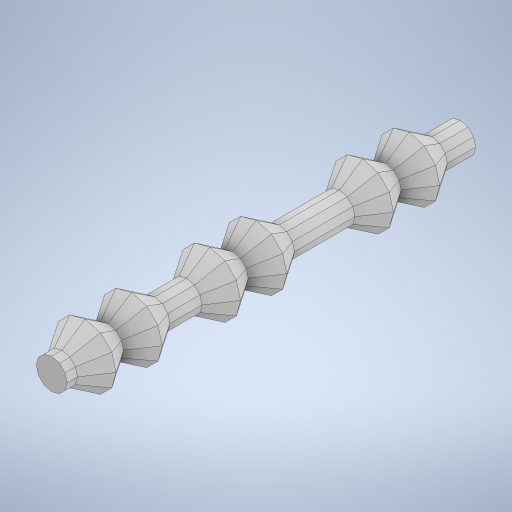
# Autodesk Inventor part: Finger
Saved by Autodesk Inventor 2023 (Build 270158000, 158)
## iProperties
Created: 2024-07-10
Part Number: Finger
Material: 일반
Document SubType Name: Modeling
Designer: ojs08
Density: 1 g/cm^3
Appearance: 기본값
Author: ojs08
Autodesk Inventor part; units mm, degrees
sketch "스케치1" plane through (0, 0, 0) normal (0, 0, 1) x (1, 0, 0)
  line L0 (6, -10.392305) -> (0, -12)
  line L1 (0, -12) -> (-6, -10.392305)
  line L2 (-6, -10.392305) -> (-10.392305, -6)
  line L3 (-10.392305, -6) -> (-12, 0)
  line L4 (-12, 0) -> (-10.392305, 6)
  line L5 (-10.392305, 6) -> (-6, 10.392305)
  line L6 (-6, 10.392305) -> (0, 12)
  line L7 (0, 12) -> (6, 10.392305)
  line L8 (6, 10.392305) -> (10.392305, 6)
  line L9 (10.392305, 6) -> (12, 0)
  line L10 (12, 0) -> (10.392305, -6)
  line L11 (10.392305, -6) -> (6, -10.392305)
  line L12 (-16.8, 0) -> (16.8, 0)
  point P0 (0, 0)
  point P1 (0, 0)
  dimension "d0" = 24
  constraints: 24 end point, 1 coincident, 1 point on line, 25 other
  measures "d0" distance of L9.end L3.end
ref_plane "작업 평면1" through (0, 0, 9) normal (0, 0, 1) x (1, 0, 0)
sketch "스케치2" plane through (0, 0, 9) normal (0, 0, 1) x (1, 0, 0)
  line L0 (-16.8, 0) -> (16.8, 0)
  line L1 (5.196152, -3) -> (3, -5.196152)
  line L2 (3, -5.196152) -> (0, -6)
  line L3 (0, -6) -> (-3, -5.196152)
  line L4 (-3, -5.196152) -> (-5.196152, -3)
  line L5 (-5.196152, -3) -> (-6, 0)
  line L6 (-6, 0) -> (-5.196152, 3)
  line L7 (-5.196152, 3) -> (-3, 5.196152)
  line L8 (-3, 5.196152) -> (0, 6)
  line L9 (0, 6) -> (3, 5.196152)
  line L10 (3, 5.196152) -> (5.196152, 3)
  line L11 (5.196152, 3) -> (6, 0)
  line L12 (6, 0) -> (5.196152, -3)
  point P0 (0, 0)
  point P1 (0, 0)
  dimension "d2" = 12
  constraints: 24 end point, 1 coincident, 1 point on line, 25 other
  measures "d2" distance of L11.end L5.end
loft "로프트1" add profiles "스케치2", "스케치1"
mirror "미러1" about plane through (0, 0, 0) normal (0, 0, -1) of "로프트1"
mirror "미러2" about plane through (0, 0, 9) normal (0, 0, 1) of "로프트1", "미러1"
sketch "스케치3" plane through (3, -5.196152, 27) normal (0, 0, 1) x (0.7071068, -0.7071068, 0)
  line L0 (0, 3.105829) -> (0, 0)
  line L1 (-1.552914, 5.795555) -> (0, 3.105829)
  line L2 (-4.242641, 7.348469) -> (-1.552914, 5.795555)
  line L3 (-7.348469, 7.348469) -> (-4.242641, 7.348469)
  line L4 (-10.038196, 5.795555) -> (-7.348469, 7.348469)
  line L5 (-11.59111, 3.105829) -> (-10.038196, 5.795555)
  line L6 (-11.59111, 0) -> (-11.59111, 3.105829)
  line L7 (-10.038196, -2.689726) -> (-11.59111, 0)
  line L8 (-7.348469, -4.242641) -> (-10.038196, -2.689726)
  line L9 (-4.242641, -4.242641) -> (-7.348469, -4.242641)
  line L10 (-1.552914, -2.689726) -> (-4.242641, -4.242641)
  line L11 (0, 0) -> (-1.552914, -2.689726)
  point P0 (-5.795555, 1.552914)
extrude "돌출1" add sketch "스케치3" along normal blind 23.5
ref_plane "작업 평면2" through (3, -5.196152, 38.75) normal (0, 0, 1) x (0.7071068, 0.7071068, 0)
mirror "미러3" about plane through (3, -5.196152, 38.75) normal (0, 0, 1) of "로프트1", "미러1", "미러2"
sketch "스케치4" plane through (3, -5.196152, 86.5) normal (0, 0, 1) x (0.7071068, -0.7071068, 0)
  line L0 (0, 3.105829) -> (0, 0)
  line L1 (-1.552914, 5.795555) -> (0, 3.105829)
  line L2 (-4.242641, 7.348469) -> (-1.552914, 5.795555)
  line L3 (-7.348469, 7.348469) -> (-4.242641, 7.348469)
  line L4 (-10.038196, 5.795555) -> (-7.348469, 7.348469)
  line L5 (-11.59111, 3.105829) -> (-10.038196, 5.795555)
  line L6 (-11.59111, 0) -> (-11.59111, 3.105829)
  line L7 (-10.038196, -2.689726) -> (-11.59111, 0)
  line L8 (-7.348469, -4.242641) -> (-10.038196, -2.689726)
  line L9 (-4.242641, -4.242641) -> (-7.348469, -4.242641)
  line L10 (-1.552914, -2.689726) -> (-4.242641, -4.242641)
  line L11 (0, 0) -> (-1.552914, -2.689726)
  point P0 (-5.795555, 1.552914)
extrude "돌출2" add sketch "스케치4" along normal blind 12.5
ref_plane "작업 평면6" through (3, -5.196152, 63) normal (0, 0, 1) x (0.7071068, 0.7071068, 0)
mirror "미러5" about plane through (3, -5.196152, 63) normal (0, 0, 1) of "로프트1", "미러1", "미러2"
sketch "스케치5" plane through (3, -5.196152, -9) normal (0, 0, -1) x (-0.7071068, 0.7071068, 0)
  line L0 (0, 3.105829) -> (0, 0)
  line L1 (0, 0) -> (1.552914, -2.689726)
  line L2 (1.552914, -2.689726) -> (4.242641, -4.242641)
  line L3 (4.242641, -4.242641) -> (7.348469, -4.242641)
  line L4 (7.348469, -4.242641) -> (10.038196, -2.689726)
  line L5 (10.038196, -2.689726) -> (11.59111, 0)
  line L6 (11.59111, 0) -> (11.59111, 3.105829)
  line L7 (11.59111, 3.105829) -> (10.038196, 5.795555)
  line L8 (10.038196, 5.795555) -> (7.348469, 7.348469)
  line L9 (7.348469, 7.348469) -> (4.242641, 7.348469)
  line L10 (4.242641, 7.348469) -> (1.552914, 5.795555)
  line L11 (1.552914, 5.795555) -> (0, 3.105829)
  point P0 (5.795555, 1.552914)
extrude "돌출3" add sketch "스케치5" along normal blind 7.5
shell "쉘1" thickness 0.5 removed faces 0 ; own thickness 2 on faces at (10.26314, 2.75, 1.5) (7.51314, 7.51314, 1.5) (2.75, 10.26314, 1.5) (-2.75, 10.26314, 1.5) (-7.51314, 7.51314, 1.5) (-10.26314, -2.75, 1.5) (-10.26314, 2.75, 1.5) (10.26314, -2.75, 1.5) (7.51314, -7.51314, 1.5) (2.75, -10.26314, 1.5) (-2.75, -10.26314, 1.5) (-7.51314, -7.51314, 1.5) (-10.26314, -2.75, 19.5) (-7.51314, -7.51314, 19.5) (-2.75, -10.26314, 19.5) (2.75, -10.26314, 19.5) (7.51314, -7.51314, 19.5) (10.26314, -2.75, 19.5) (10.26314, 2.75, 19.5) (7.51314, 7.51314, 19.5) (2.75, 10.26314, 19.5) (-2.75, 10.26314, 19.5) (-7.51314, 7.51314, 19.5) (-10.26314, 2.75, 19.5) (-5.464102, 2, 34.833333) (-3.732051, 4.464102, 34.833333) (-1, 5.732051, 42.666667) (2, 5.464102, 34.833333) (4.464102, 3.732051, 34.833333) (5.732051, 1, 34.833333) (5.464102, -2, 34.833333) (4.464102, -3.732051, 42.666667) (-5.732051, -1, 42.666667) (-4.464102, -3.732051, 34.833333) (-2, -5.464102, 34.833333) (1, -5.732051, 34.833333) (-2.75, -10.26314, 61) (2.75, -10.26314, 61) (7.51314, -7.51314, 61) (10.26314, -2.75, 61) (10.26314, 2.75, 61) (7.51314, 7.51314, 61) (2.75, 10.26314, 61) (-2.75, 10.26314, 61) (-7.51314, 7.51314, 61) (-7.51314, -7.51314, 61) (-10.26314, -2.75, 61) (-10.26314, 2.75, 61) (-7.51314, -7.51314, 79) (-2.75, -10.26314, 79) (2.75, -10.26314, 79) (7.51314, -7.51314, 79) (10.26314, -2.75, 79) (10.26314, 2.75, 79) (7.51314, 7.51314, 79) (2.75, 10.26314, 79) (-2.75, 10.26314, 79) (-7.51314, 7.51314, 79) (-10.26314, 2.75, 79) (-10.26314, -2.75, 79) (-5.464102, 2, 90.666667) (-5.732051, -1, 90.666667) (-4.464102, -3.732051, 94.833333) (-2, -5.464102, 90.666667) (2, 5.464102, 90.666667) (1, -5.732051, 90.666667) (4.464102, 3.732051, 90.666667) (5.732051, 1, 90.666667) (5.464102, -2, 90.666667) (4.464102, -3.732051, 94.833333) (-1, 5.732051, 90.666667) (-3.732051, 4.464102, 90.666667) (-2.75, -10.26314, 109.5) (2.75, -10.26314, 109.5) (7.51314, -7.51314, 109.5) (10.26314, -2.75, 109.5) (10.26314, 2.75, 109.5) (7.51314, 7.51314, 109.5) (2.75, 10.26314, 109.5) (-2.75, 10.26314, 109.5) (-7.51314, 7.51314, 109.5) (-10.26314, 2.75, 109.5) (-10.26314, -2.75, 109.5) (-7.51314, -7.51314, 109.5) (-2.75, -10.26314, 127.5) (2.75, -10.26314, 127.5) (7.51314, -7.51314, 127.5) (10.26314, -2.75, 127.5) (10.26314, 2.75, 127.5) (7.51314, 7.51314, 127.5) (2.75, 10.26314, 127.5) (-2.75, 10.26314, 127.5) (-7.51314, 7.51314, 127.5) (-10.26314, 2.75, 127.5) (-10.26314, -2.75, 127.5) (-7.51314, -7.51314, 127.5) (5.464102, -2, -14) (4.464102, -3.732051, -11.5) (1, -5.732051, -14) (-1, -5.732051, -11.5) (3.732051, 4.464102, -14) (5.464102, 2, -11.5) (1, 5.732051, -11.5) (-5.464102, -2, -11.5) (-4.464102, -3.732051, -14) (-5.732051, 1, -11.5) (-3.732051, 4.464102, -14) (-1, 5.732051, -14)
sketch "스케치6" plane through (3, -5.196152, -16.5) normal (0, 0, -1) x (-0.7071068, -0.7071068, 0)
  line L0 (0, 0) -> (2.689726, 1.552914)
  line L1 (2.689726, 1.552914) -> (4.242641, 4.242641)
  line L2 (4.242641, 4.242641) -> (4.242641, 7.348469)
  line L3 (4.242641, 7.348469) -> (2.689726, 10.038196)
  line L4 (2.689726, 10.038196) -> (0, 11.59111)
  line L5 (0, 11.59111) -> (-3.105829, 11.59111)
  line L6 (-3.105829, 11.59111) -> (-5.795555, 10.038196)
  line L7 (-5.795555, 10.038196) -> (-7.348469, 7.348469)
  line L8 (-7.348469, 7.348469) -> (-7.348469, 4.242641)
  line L9 (-7.348469, 4.242641) -> (-5.795555, 1.552914)
  line L10 (-5.795555, 1.552914) -> (-3.105829, 0)
  line L11 (-3.105829, 0) -> (0, 0)
  point P0 (-1.552914, 5.795555)
extrude "돌출4" add sketch "스케치6" along normal blind 3.5
sketch "스케치7" plane through (3, -5.196152, -20) normal (0, 0, -1) x (-0.7071068, 0.7071068, 0)
  circle A0 centre (5.795555, 1.552914) radius 2.25
  dimension "d21" = 4.5
  constraints: 1 centre point, 1 coincident
  measures "d21" diameter of A0
extrude "돌출5" cut sketch "스케치7" against normal blind 4
sketch "스케치8" plane through (3, -5.196152, 135) normal (0, 0, 1) x (0.7071068, -0.7071068, 0)
  line L0 (0, 3.105829) -> (0, 0)
  line L1 (-1.552914, 5.795555) -> (0, 3.105829)
  line L2 (-4.242641, 7.348469) -> (-1.552914, 5.795555)
  line L3 (-7.348469, 7.348469) -> (-4.242641, 7.348469)
  line L4 (-10.038196, 5.795555) -> (-7.348469, 7.348469)
  line L5 (-11.59111, 3.105829) -> (-10.038196, 5.795555)
  line L6 (-11.59111, 0) -> (-11.59111, 3.105829)
  line L7 (-10.038196, -2.689726) -> (-11.59111, 0)
  line L8 (-7.348469, -4.242641) -> (-10.038196, -2.689726)
  line L9 (-4.242641, -4.242641) -> (-7.348469, -4.242641)
  line L10 (-1.552914, -2.689726) -> (-4.242641, -4.242641)
  line L11 (0, 0) -> (-1.552914, -2.689726)
  point P0 (-5.795555, 1.552914)
extrude "돌출6" add sketch "스케치8" along normal blind 4
